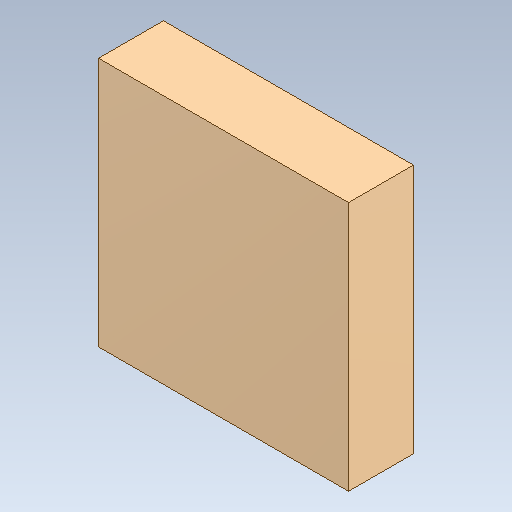
# Autodesk Inventor part: TPS6300
Saved by Autodesk Inventor 2021 (Build 250183000, 183)
## iProperties
Created: 2020-11-03
Part Number: TPS6300
Material: Generic
Document SubType Name: Modeling
Designer: faiya
Density: 1 g/cm^3
Appearance: DRC-S-PVSON-N10, TPS6300
Author: faiya
Autodesk Inventor part; units mm, degrees
ref_plane "YZ Plane" through (0, 0, 0) normal (1, 0, 0) x (0, 1, 0)
ref_plane "XZ Plane" through (0, 0, 0) normal (0, 1, 0) x (-1, 0, 0)
ref_plane "XY Plane" through (0, 0, 0) normal (0, 0, 1) x (1, 0, 0)
sketch "DRC-S-PVSON-N10, TPS6300_46" plane through (0, 0, 0) normal (0, 0, 1) x (1, 0, 0)
  line L0 (-1.925, 1.925) -> (1.925, 1.925)
  line L1 (1.925, 1.925) -> (1.925, -1.925)
  line L2 (1.925, -1.925) -> (-1.925, -1.925)
  line L3 (-1.925, -1.925) -> (-1.925, 1.925)
  constraints: 8 end point
extrude "Extrusion1" add sketch "DRC-S-PVSON-N10, TPS6300_46" along normal blind 1
body "Solid1"
